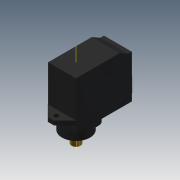
# Autodesk Inventor part: Servo ES08MA2
Saved by Autodesk Inventor 2018 (Build 220112000, 112)
## iProperties
Created: 2013-10-15
Part Number: Servo ES08MA2
Material: ABS-Kunststoff - Schwarz
Document SubType Name: Modeling
Designer: 4ndreas
Density: 1.06 g/cm^3
Appearance: Glatt - weiß(2)
Mass: 7.06899 g
Surface Area: 25.6588 cm^2
Volume: 6.66886 cm^3
Author: 4ndreas
Autodesk Inventor part; units mm, degrees
ref_plane "YZ Plane" through (0, 0, 0) normal (1, 0, 0) x (0, 1, 0)
ref_plane "XZ Plane" through (0, 0, 0) normal (0, 1, 0) x (-1, 0, 0)
ref_plane "XY Plane" through (0, 0, 0) normal (0, 0, 1) x (1, 0, 0)
sketch "Skizze1" plane through (0, 0, 0) normal (0, 0, 1) x (1, 0, 0)
  line L0 (5.75, 11.5) -> (5.75, -11.5)
  line L1 (5.75, -11.5) -> (-5.75, -11.5)
  line L2 (-5.75, -11.5) -> (-5.75, 11.5)
  line L3 (-5.75, 11.5) -> (5.75, 11.5)
  line L4 (5.75, -11.5) -> (-5.75, 11.5) construction
  line L5 (-5.75, -11.5) -> (5.75, 11.5) construction
  point P0 (0, 0)
  point P1 (0, 0)
  point P2 (0, 0)
  point P3 (0, 0)
  dimension "d34" = 11.5
  dimension "d35" = 23
  constraints: 12 end point, 2 coincident, 2 midpoint, 1 perpendicular
  measures "d34" distance between parallel lines of L0 L2
  measures "d35" distance between parallel lines of L1 L3
extrude "Extrusion1" add sketch "Skizze1" against normal blind 3
sketch "Skizze2" plane through (0, 0, 0) normal (0, 0, 1) x (1, 0, 0)
  line L0 (5.75, 11.5) -> (-5.75, 11.5) projected
  line L1 (-5.75, -11.5) -> (5.75, -11.5) projected
  line L2 (-5.75, 16.1) -> (5.75, 16.1)
  line L3 (5.75, 16.1) -> (5.75, 11.5)
  line L4 (5.75, -16.1) -> (-5.75, -16.1)
  line L5 (-5.75, -16.1) -> (-5.75, -11.5)
  line L6 (5.75, -11.5) -> (5.75, -16.1)
  line L7 (-5.75, 11.5) -> (-5.75, 16.1)
  point P0 (0, 0)
  dimension "d58" = 32.2
  constraints: 16 end point, 5 parallel, 2 perpendicular, 1 collinear, 1 horizontal
  measures "d58" distance between parallel lines of L2 L4
extrude "Extrusion2" add sketch "Skizze2" along normal blind 1.7
sketch "Skizze3" plane through (0, 0, 1.7) normal (0, 0, 1) x (1, 0, 0)
  line L0 (5.75, 11.5) -> (5.75, -11.5) projected
  line L1 (5.75, -11.5) -> (-5.75, -11.5) projected
  line L2 (-5.75, -11.5) -> (-5.75, 11.5) projected
  line L3 (-5.75, 11.5) -> (5.75, 11.5) projected
  point P0 (0, 0)
extrude "Extrusion3" add sketch "Skizze3" along normal blind 15 and the other way blind 2
sketch "Skizze4" plane through (0, 0, -3) normal (0, 0, -1) x (-1, 0, 0)
  line L0 (-5.75, -11.5) -> (5.75, -11.5) projected
  line L1 (5.75, 11.5) -> (-5.75, 11.5) projected
  circle A0 centre (0, -5.75) radius 5.75
  line L2 (0, 11.5) -> (0, -11.5) construction
  line L3 (0, -5.75) -> (0, 0.25) construction
  line L4 (3.25, -5.75) -> (3.25, 0.25)
  line L5 (-3.25, 0.25) -> (-3.25, -5.75)
  arc A1 (-3.25, -5.75) -> (3.25, -5.75) centre (0, -5.75) ccw
  arc A2 (3.25, 0.25) -> (-3.25, 0.25) centre (0, 0.25) ccw
  line L6 (-5.75, 11.5) -> (-5.75, -11.5) projected
  point P0 (0, 0)
  point P1 (0, -2.75)
  dimension "d32" = 6.5
  dimension "d33" = 15
  constraints: 10 end point, 6 tangent, 4 point on circle, 3 centre point, 3 midpoint, 2 point on line, 1 parallel
  measures "d32" distance between parallel lines of L4 L5
extrude "Extrusion4" add sketch "Skizze4" along normal blind 4.3 contours A0 L5 A1 L4 | L5 A2 L4 A0 | A0 L4 A1 L5
sketch "Skizze5" plane through (0, 0, -3) normal (0, 0, -1) x (-1, 0, 0)
  circle A0 centre (0, -5.75) radius 5.75 projected
  line L0 (-5.75, 11.5) -> (-5.75, -11.5) projected
  line L1 (-5.75, -11.5) -> (5.75, -11.5) projected
  line L2 (5.75, -11.5) -> (5.75, 11.5) projected
  line L3 (5.75, 11.5) -> (-5.75, 11.5) projected
  point P0 (0, 0)
sketch "Skizze7" plane through (0, 0, 0) normal (0, 0, -1) x (-1, 0, 0)
  line L0 (0, -11.5) -> (5.75, -11.5) projected
  line L1 (-5.75, -11.5) -> (5.75, -11.5) projected
  line L2 (-8.05, 0) -> (8.05, 0) construction
  point P0 (0, 0)
  point P1 (0, -13.8)
  point P2 (0, 13.8)
  dimension "d59" = 27.6
  constraints: 1 symmetric about line
  measures "d59" distance of point (0, 13.8) point (0, -13.8)
hole "Bohrung1" at (0, -13.8, 0) at (0, 13.8, 0) direction (0, 0, 1) diameter 1.7 end through all
sketch "Skizze9" plane through (0, 0, -7.3) normal (0, 0, -1) x (-1, 0, 0)
  arc A0 (-3.25, -1.0066) -> (3.25, -1.0066) centre (0, -5.75) ccw projected
  circle A1 centre (0, -5.75) radius 1.85
  point P0 (0, 0)
  dimension "d36" = 3.7
  constraints: 1 centre point, 1 coincident
  measures "d36" diameter of A1
extrude "Extrusion6" add sketch "Skizze9" along normal blind 5 separate body
chamfer "Fase1" distance 0.2 angle 45 1 edges at (1.85, -5.75, -12.3)
sketch "Skizze10" plane through (5.75, 11.5, 0) normal (1, 0, 0) x (0, 0, -1)
  line L0 (-1.7, 0) -> (-16.7, 0) projected
  line L1 (-16.7, -23) -> (-16.7, 0) projected
  line L2 (0, 4.6) -> (0, -27.6) projected
  line L3 (-14.7, 0) -> (-14.7, -1.5359)
  line L4 (-14.7, -1.5359) -> (-16.7, -5)
  point P0 (0, -23)
  point P1 (0, -11.5)
  point P2 (1.7, 0)
  dimension "d42" = 30
  dimension "d43" = 2
  dimension "d44" = 5
  constraints: 4 end point, 2 point on line, 1 parallel
  measures "d42" angle of L1 L4
  measures "d43" distance between parallel lines of L1 L3
  measures "d44" distance from line of L4.end L0
extrude "Extrusion7" cut sketch "Skizze10" against normal through all bodies 1
hole "Bohrung2" at (0, -5.75, -12.3) direction (0, 0, 1) diameter 2 depth 5 tip angle 118 bodies 2
chamfer "Chamfer2" distance 4.5 angle 45 4 edges at (-5.75, -16.1, 0.85) (5.75, -16.1, 0.85) (-5.75, 16.1, 0.85) (5.75, 16.1, 0.85)
